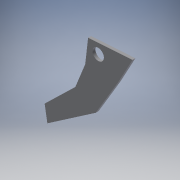
# Autodesk Inventor part: Leg
Saved by Autodesk Inventor 2016 (Build 200138000, 138)
## iProperties
Created: 2015-10-16
Part Number: Leg
Material: Generic
Document SubType Name: Modeling
Designer: powasar16
Density: 1 g/cm^3
Appearance: Default
Author: powasar16
Autodesk Inventor part; units mm, degrees
ref_plane "YZ Plane" through (0, 0, 0) normal (1, 0, 0) x (0, 1, 0)
ref_plane "XZ Plane" through (0, 0, 0) normal (0, 1, 0) x (-1, 0, 0)
ref_plane "XY Plane" through (0, 0, 0) normal (0, 0, 1) x (1, 0, 0)
sketch "Sketch1" plane through (0, 0, 0) normal (0, 0, 1) x (1, 0, 0)
  circle A0 centre (2.8854, -1.4956) radius 3.75 projected
  line L0 (25.3345, 6.5712) -> (-3.7329, 4.6517)
  line L1 (-3.7329, 4.6517) -> (-5.6525, -11.3903)
  line L2 (-5.6525, -11.3903) -> (-12.1454, -27.5582)
  line L3 (-12.1454, -27.5582) -> (-32.252, -47.0391)
  line L4 (-32.252, -47.0391) -> (-30.4695, -57.3224)
  line L5 (-30.4695, -57.3224) -> (1.203, -35.5218)
  line L6 (1.203, -35.5218) -> (15.5997, -11.3903)
  line L7 (15.5997, -11.3903) -> (25.3345, 6.5712)
  point P0 (0, 0)
  constraints: 16 end point
extrude "Extrusion1" add sketch "Sketch1" along normal blind 1.905
body "Solid1"
